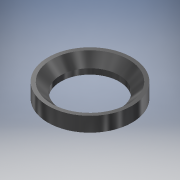
# Autodesk Inventor part: Bumper
Saved by Autodesk Inventor 2018 (Build 220112000, 112)
## iProperties
Shininess: 64.0
Length Units: 11269
Angle Units: 11279
Time Units: 11290
Mass Units: 11283
Length Display Precision: 3
Angle Display Precision: 2
Compacted: True
Part Number: Bumper
Document SubType Name: Modeling
Created: 2003-04-19
Designer: James M. Leake
Material: Silicone
Density: 1.25 g/cm^3
Appearance: Rubber - Black - Version 1.1
Density: 0.0
Volumn: 0.0
Area: 0.0
PropertySet Name: Model Information
Control State: 0
Master: False
Checked Out: False
Author: James M. Leake
Autodesk Inventor part; units mm, degrees
ref_plane "YZ Plane" through (0, 0, 0) normal (1, 0, 0) x (0, 1, 0)
ref_plane "XZ Plane" through (0, 0, 0) normal (0, 1, 0) x (-1, 0, 0)
ref_plane "XY Plane" through (0, 0, 0) normal (0, 0, 1) x (1, 0, 0)
sketch "Sketch1" plane through (0, 0, 0) normal (0, 0, 1) x (1, 0, 0)
  line L0 (-27.6, 0) -> (36.8, 0) projected
  line L1 (0, -27.6) -> (0, 36.8) projected
  circle A0 centre (0, 0) radius 23
  dimension "d0" = 46
  constraints: 1 centre point, 1 coincident
  measures "d0" diameter of A0
extrude "Extrusion1" add sketch "Sketch1" along normal blind 8
sketch "Sketch3" plane through (0, 0, 8) normal (0, 0, 1) x (1, 0, 0)
  circle A0 centre (0, 0) radius 23 projected
  constraints: 1 coincident
hole "Hole1" at (0, 0, 8) direction (0, 0, -1) diameter 32 end through all
chamfer "Chamfer1" distance 5 angle 45 1 edges at (0, 16, 8)
body "Solid1"
